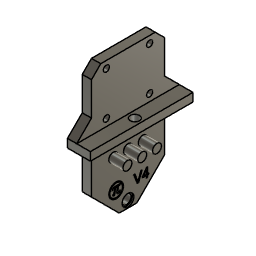
3. BLDC motor holder [V4] (Autodesk Fusion 360 design; units mm, degrees)
Autodesk Fusion 360 part; units mm, degrees
sketch "Base" plane through (0, 0, 0) normal (0, 0, 1) x (1, 0, 0)
  line L0 (0, 0) -> (5, 0)
  line L1 (5, 0) -> (5, 39.5)
  line L2 (5, 39.5) -> (0, 39.5)
  line L3 (0, 39.5) -> (0, 0)
  dimension "d1" = 39.5
  dimension "d2" = 5
  constraint horizontal L0
  constraint vertical L1
  constraint horizontal L2
  constraint vertical L3
  constraint coincident L0.start L3.end
  measures "d1" distance of L0.start L2.end
  measures "d2" distance of L0.start L0.end
extrude "Extrude1" add sketch "Base" along normal blind 39.5 makes body 1
sketch "Bottom round hole" plane through (5, 0, 0) normal (1, 0, 0) x (0, 1, 0)
  circle A0 centre (19.75, 3.7) radius 3.7
  line L0 (0, 0) -> (0, 39.5)
  line L1 (39.5, 0) -> (39.5, 39.5)
  line L2 (39.5, 0) -> (0, 0)
  circle A1 centre (19.75, 3.7) radius 3.2
  circle A2 centre (19.75, 3.7) radius 2.5
  line L3 (0, 0) -> (39.5, 0)
  line L4 (39.5, 0) -> (39.5, 39.5)
  line L5 (39.5, 39.5) -> (0, 39.5)
  line L6 (0, 39.5) -> (0, 0)
  line L7 (24.5, 0) -> (39.5, 15)
  line L8 (24.5, 0) -> (43.435, 0) construction
  line L9 (15, 0) -> (0, 15)
  line L10 (15, 0) -> (21.7279, 0) construction
  dimension "d5" = 19.75
  dimension "d6" = 19.75
  dimension "d7" = 7.4
  dimension "d8" = 6.4
  dimension "d9" = 5
  dimension "d73" = 45
  dimension "d74" = 135
  dimension "d75" = 15
  dimension "d76" = 15
  constraint tangent A0 L2
  constraint concentric A0 A1
  constraint concentric A0 A2
  constraint horizontal L8
  constraint coincident L2 L7.start
  constraint coincident L4 L7.end
  constraint horizontal L10
  constraint coincident L3 L9.start
  constraint coincident L0 L9.end
  measures "d5" distance of A0.centre L0
  measures "d6" distance of A0.centre L1
  measures "d7" diameter of A0
  measures "d8" diameter of A1
  measures "d9" diameter of A2
  measures "d73" angle of L7 L8
  measures "d74" angle of L9 L10
  measures "d75" distance of L1.start L7.start
  measures "d76" distance of L9.start L0.start
sketch "Middle support" plane through (0, 0, 39.5) normal (0, 0, 1) x (-1, 0, 0)
  line L0 (0, -39.5) -> (0, 0)
  line L1 (0, 0) -> (-5, 0)
  line L2 (-5, 0) -> (-5, -39.5)
  line L3 (-5, -39.5) -> (0, -39.5)
  line L4 (0, 8) -> (-13.9, 8)
  line L5 (-13.9, 8) -> (-13.9, -47.5)
  line L6 (-13.9, -47.5) -> (0, -47.5)
  line L7 (0, -47.5) -> (0, 8)
  line L8 (0, 0) -> (-13.9, 0)
  line L9 (-13.9, 0) -> (-13.9, -8)
  line L10 (-13.9, -8) -> (0, -8)
  line L11 (0, -8) -> (0, 0)
  line L12 (0, -39.5) -> (-13.9, -39.5)
  line L13 (-13.9, -39.5) -> (-13.9, -31.5)
  line L14 (-13.9, -31.5) -> (0, -31.5)
  line L15 (0, -31.5) -> (0, -39.5)
  line L16 (0, -39.5) -> (-6.5, -39.5)
  line L17 (-6.5, -39.5) -> (-6.5, -47.5)
  line L18 (-6.5, -47.5) -> (0, -47.5)
  line L19 (0, -47.5) -> (0, -39.5)
  line L20 (0, 0) -> (-6.5, 0)
  line L21 (-6.5, 0) -> (-6.5, 8)
  line L22 (-6.5, 8) -> (0, 8)
  line L23 (0, 8) -> (0, 0)
  dimension "d10" = 13.9
  dimension "d11" = 8
  dimension "d12" = 8
  dimension "d13" = 8
  dimension "d14" = 8
  constraint horizontal L4
  constraint vertical L5
  constraint horizontal L6
  constraint vertical L7
  constraint horizontal L8
  constraint vertical L9
  constraint horizontal L10
  constraint vertical L11
  constraint coincident L5 L9.end
  constraint coincident L0.end L1.start
  constraint horizontal L12
  constraint vertical L13
  constraint horizontal L14
  constraint vertical L15
  constraint coincident L5 L13.end
  constraint coincident L0.start L3.end
  constraint horizontal L16
  constraint vertical L17
  constraint horizontal L18
  constraint vertical L19
  constraint coincident L6 L17.end
  constraint horizontal L20
  constraint vertical L21
  constraint horizontal L22
  constraint vertical L23
  constraint coincident L4 L21.end
  measures "d10" distance of L4.start L4.end
  measures "d11" distance of L3 L6
  measures "d12" distance of L1 L4
  measures "d13" distance of L0.end L10.end
  measures "d14" distance of L0.start L14.end
extrude "Extrude4" add sketch "Middle support" along normal blind 4.5 bodies 1
extrude "Extrude5" add sketch "Middle support" along normal blind 35.5 separate body contours L0 L2 L3 L7 L12 L14 L15 L16 | L0 L2 L7 L10 L14 | L0 L1 L2 L7 L8 L10 L11 L20 makes body 2
sketch "Motor round holes" plane through (5, 0, 0) normal (1, 0, 0) x (0, 1, 0)
  line L0 (0, 39.5) -> (39.5, 39.5)
  line L1 (39.5, 75) -> (0, 75)
  line L2 (19.75, 42.5167) -> (19.75, 75)
  circle A0 centre (8.05, 47.8) radius 3.8
  line L3 (-8, 44) -> (47.5, 44)
  circle A1 centre (8.05, 47.8) radius 1.65
  line L4 (47.5, 44) -> (0, 44)
  line L5 (0, 44) -> (0, 75)
  line L6 (0, 59.5) -> (39.5, 59.5)
  circle A2 centre (8.05, 71.2) radius 1.65
  circle A3 centre (8.05, 71.2) radius 3.8
  circle A4 centre (31.45, 71.2) radius 3.8
  circle A5 centre (31.45, 71.2) radius 1.65
  circle A6 centre (31.45, 47.8) radius 3.8
  circle A7 centre (31.45, 47.8) radius 1.65
  line L7 (39.5, 39.5) -> (39.5, 75)
  line L8 (0, 75) -> (0, 39.5)
  line L9 (0, 75) -> (39.5, 75)
  line L10 (39.5, 75) -> (39.4892, 44)
  dimension "d23" = 11.7
  dimension "d24" = 7.6
  dimension "d25" = 3.3
  constraint midpoint L1 L2.end
  constraint perpendicular L1 L2
  constraint tangent A0 L3
  constraint concentric A0 A1
  constraint horizontal L4
  constraint vertical L5
  constraint coincident L3.end L4.start
  constraint coincident L1.end L5.end
  constraint midpoint L5 L6.start
  constraint symmetric A0 L6 A3
  constraint symmetric A1 L6 A2
  constraint symmetric L2 A0 A6
  constraint symmetric L2 A1 A7
  constraint symmetric L2 A2 A5
  constraint symmetric L2 A3 A4
  constraint coincident L1.start L7.end
  constraint coincident L4 L10.end
  constraint coincident L6.end L7
  constraint perpendicular L6 L7
  measures "d23" distance of L2 A0.centre
  measures "d24" diameter of A0
  measures "d25" diameter of A1
sketch "Middle top round hole" plane through (0, 0, 39.5) normal (0, 0, 1) x (-1, 0, 0)
  line L0 (-5, -8) -> (-12.4, -8)
  line L1 (-12.4, -8) -> (-12.4, -31.5)
  line L2 (-12.4, -31.5) -> (-5, -31.5)
  line L3 (-5, -31.5) -> (-5, -8)
  line L4 (-12.4, -19.75) -> (-5, -19.75)
  line L5 (-8.7, -8) -> (-8.7, -31.5)
  circle A0 centre (-8.7, -19.75) radius 3.2
  circle A1 centre (-8.7, -19.75) radius 2.5
  dimension "d26" = 6.4
  dimension "d27" = 5
  constraint horizontal L0
  constraint vertical L1
  constraint horizontal L2
  constraint vertical L3
  constraint midpoint L1 L4.start
  constraint midpoint L3 L4.end
  constraint midpoint L0 L5.start
  constraint midpoint L2 L5.end
  constraint midpoint L4 A0.centre
  constraint concentric A0 A1
  measures "d26" diameter of A0
  measures "d27" diameter of A1
extrude "Extrude6" cut sketch "Middle top round hole" along normal blind 5 contours L4 L5 A1 | L4 L5 A1 | L4 L5 A1 | L4 L5 A1 bodies 1
extrude "Extrude7" cut sketch "Middle top round hole" along normal blind 0.8 contours L4 L5 A0 A1 | L4 L5 A0 A1 | L4 L5 A0 A1 | L4 L5 A0 A1 bodies 1
extrude "Extrude8" cut sketch "Motor round holes" against normal blind 7 contours A1 | A2 | A5 | A7 bodies 2
extrude "Extrude9" cut sketch "Bottom round hole" against normal blind 10 contours A2 bodies 1
extrude "Extrude10" cut sketch "Bottom round hole" against normal blind 0.8 contours A1 bodies 1
extrude "Extrude11" add 1 faces at (4.2, 22.6954, 3.4168) along direction (-1, 0, 0) blind 6.1 on bodies 1 bodies 1
extrude "Extrude12" add sketch "Bottom round hole" against normal blind 7.7 contours A0 bodies 1
sketch "Motor rest area support" plane through (0, 0, 0) normal (-1, 0, 0) x (0, -1, 0)
  circle A0 centre (-31.45, 71.2) radius 1.65
  circle A1 centre (-8.05, 47.8) radius 1.65
  circle A2 centre (-8.05, 71.2) radius 1.65
  circle A3 centre (-31.45, 47.8) radius 1.65
  line L0 (-39.5, 39.5) -> (0, 39.5)
  line L1 (0, 39.5) -> (0, 75)
  line L2 (0, 75) -> (-39.5, 75)
  line L3 (-39.5, 75) -> (-39.5, 39.5)
  line L4 (-47.5, 44) -> (-39.5, 52)
  line L5 (-47.5, 44) -> (-36.1863, 44) construction
  line L6 (8, 44) -> (0, 52)
  line L7 (8, 44) -> (19.3137, 44) construction
  line L8 (0, 52) -> (8, 52)
  line L9 (8, 52) -> (8, 44)
  line L10 (8, 44) -> (0, 44)
  line L11 (0, 44) -> (0, 52)
  line L12 (-39.5, 52) -> (-47.5, 52)
  line L13 (-47.5, 52) -> (-47.5, 44)
  line L14 (-47.5, 44) -> (-39.5, 44)
  line L15 (-39.5, 44) -> (-39.5, 52)
  line L16 (-5, 75) -> (0, 70)
  line L17 (-5, 75) -> (2.4834, 75) construction
  line L18 (-34.5, 75) -> (-39.5, 70)
  line L19 (-34.5, 75) -> (-27.8923, 75) construction
  dimension "d42" = 45
  dimension "d43" = 135
  dimension "d67" = 45
  dimension "d68" = 5
  dimension "d69" = 135
  dimension "d70" = 5
  constraint horizontal L5
  constraint coincident L3 L4.end
  constraint horizontal L7
  constraint coincident L1 L6.end
  constraint horizontal L8
  constraint vertical L9
  constraint horizontal L10
  constraint vertical L11
  constraint horizontal L12
  constraint vertical L13
  constraint horizontal L14
  constraint vertical L15
  constraint horizontal L17
  constraint coincident L2 L16.start
  constraint coincident L1 L16.end
  constraint horizontal L19
  constraint coincident L2 L18.start
  constraint coincident L3 L18.end
  measures "d42" angle of L4 L5
  measures "d43" angle of L6 L7
  measures "d67" angle of L16 L17
  measures "d68" distance of L1.end L16.start
  measures "d69" angle of L18 L19
  measures "d70" distance of L2.end L18.start
extrude "Extrude13" add sketch "Motor rest area support" against normal blind 5 contours L3 L4 L14 L15 | L1 L6 L10 L11 bodies 1 2
sketch "Middle round holes" plane through (5, 0, 0) normal (1, 0, 0) x (0, 1, 0)
  circle A0 centre (19.75, 3.7) radius 3.2
  line L0 (0, 0) -> (39.5, 0)
  line L1 (39.5, 0) -> (39.5, 39.5)
  line L2 (39.5, 39.5) -> (0, 39.5)
  line L3 (0, 39.5) -> (0, 0)
  line L4 (0, 31.5) -> (39.5, 31.5) construction
  line L5 (0, 24.1) -> (39.5, 24.1) construction
  line L6 (19.75, 31.5) -> (19.75, 24)
  line L7 (19.75, 27.75) -> (39.5, 27.75)
  line L8 (19.75, 27.75) -> (0, 27.75)
  circle A1 centre (19.75, 27.75) radius 2.425
  circle A2 centre (19.75, 27.75) radius 3.2
  circle A3 centre (27.75, 27.75) radius 2.425
  circle A4 centre (27.75, 27.75) radius 3.2
  circle A5 centre (11.75, 27.75) radius 2.425
  circle A6 centre (11.75, 27.75) radius 3.2
  dimension "d46" = 8
  dimension "d47" = 7.4
  dimension "d48" = 6.4
  dimension "d49" = 4.85
  dimension "d52" = 8
  dimension "d53" = 0
  dimension "d56" = -8
  dimension "d57" = 0
  constraint coincident L3 L4.start
  constraint coincident L1 L4.end
  constraint perpendicular L1 L4
  constraint coincident L1 L5.end
  constraint perpendicular L1 L5
  constraint midpoint L4 L6.start
  constraint perpendicular L4 L6
  constraint midpoint L6 L7.start
  constraint coincident L1 L7.end
  constraint perpendicular L1 L7
  constraint coincident L3 L8.end
  constraint perpendicular L3 L8
  constraint coincident L7.start L8.start
  constraint concentric A1 A2
  measures "d46" distance of L2 L4
  measures "d47" distance of L4 L5
  measures "d48" diameter of A2
  measures "d49" diameter of A1
extrude "Extrude14" add sketch "Middle round holes" along normal blind 7.7 contours L8 A5 | L8 A5 | L7 A3 | L7 A3 | L6 L8 A1 | L6 L8 A1 | L6 L7 A1 | L6 L7 A1 bodies 1
sketch "Author" plane through (5, 0, 0) normal (1, 0, 0) x (0, 1, 0)
  circle A0 centre (27.75, 27.75) radius 2.425
  circle A1 centre (19.75, 27.75) radius 2.425
  circle A2 centre (11.75, 27.75) radius 2.425
  circle A3 centre (19.75, 3.7) radius 3.2
  line L0 (0, 0) -> (39.5, 0)
  line L1 (39.5, 0) -> (39.5, 39.5)
  line L2 (39.5, 39.5) -> (0, 39.5)
  line L3 (0, 39.5) -> (0, 0)
  line L4 (11.1685, 12.3321) -> (11.3277, 12.3203)
  spline S0 degree 3 poles (11.3277, 12.3203) (11.4928, 12.507) (11.5577, 13.0594) (12.5307, 12.9513) knots 0 0 0 0 1 1 1 1
  spline S1 degree 3 poles (12.5307, 12.9513) (12.4953, 10.5845) (11.4574, 10.3348) (11.5223, 9.8493) knots 0 0 0 0 1 1 1 1
  spline S2 degree 3 poles (11.5223, 9.8493) (11.5459, 9.5741) (11.7641, 9.405) (12, 9.3952) knots 0 0 0 0 1 1 1 1
  spline S3 degree 3 poles (12, 9.3952) (12.745, 9.4208) (12.7116, 10.4253) (12.9435, 12.9572) knots 0 0 0 0 1 1 1 1
  line L5 (12.9435, 12.9572) -> (13.9048, 12.9572)
  spline S4 degree 3 poles (13.9048, 12.9572) (13.8537, 12.0647) (13.7141, 11.1723) (13.6984, 10.2975) knots 0 0 0 0 1 1 1 1
  spline S5 degree 3 poles (13.6984, 10.2975) (13.7102, 9.7156) (14.064, 9.405) (14.5299, 9.4011) knots 0 0 0 0 1 1 1 1
  spline S6 degree 3 poles (14.5299, 9.4011) (15.2965, 9.3756) (15.5383, 10.27) (15.5383, 10.6513) knots 0 0 0 0 1 1 1 1
  line L6 (15.5383, 10.6513) -> (15.3732, 10.6513)
  spline S7 degree 3 poles (15.3732, 10.6513) (15.3575, 10.3368) (15.2061, 10.1107) (14.8837, 10.097) knots 0 0 0 0 1 1 1 1
  spline S8 degree 3 poles (14.8837, 10.097) (14.005, 10.0852) (14.4886, 11.6421) (14.4945, 12.9454) knots 0 0 0 0 1 1 1 1
  line L7 (14.4945, 12.9454) -> (15.5383, 12.9395)
  line L8 (15.5383, 12.9395) -> (15.5324, 13.6059)
  spline S9 degree 3 poles (15.5324, 13.6059) (11.1939, 13.6269) (11.7446, 13.7119) (11.1685, 12.3321) knots 0 0 0 0 1 1 1 1
  arc A4 (9.3808, 11.5049) -> (13.3534, 15.4775) centre (13.3534, 11.5049) cw
  arc A5 (13.3534, 7.5323) -> (9.3808, 11.5049) centre (13.3534, 11.5049) cw
  arc A6 (17.326, 11.5049) -> (13.3534, 7.5323) centre (13.3534, 11.5049) cw
  arc A7 (13.3534, 15.4775) -> (17.326, 11.5049) centre (13.3534, 11.5049) cw
  arc A8 (13.3534, 14.9461) -> (13.442, 14.945) centre (13.3538, 11.5049) cw
  arc A9 (13.442, 14.945) -> (13.5306, 14.9415) centre (13.3532, 11.5049) cw
  arc A10 (13.5306, 14.9415) -> (13.619, 14.9358) centre (13.3531, 11.5049) cw
  arc A11 (13.619, 14.9358) -> (13.7072, 14.9279) centre (13.3538, 11.5049) cw
  arc A12 (13.7072, 14.9279) -> (13.7952, 14.9176) centre (13.3534, 11.5049) cw
  arc A13 (13.7952, 14.9176) -> (13.883, 14.9051) centre (13.3536, 11.5049) cw
  arc A14 (13.883, 14.9051) -> (13.9703, 14.8903) centre (13.3527, 11.505) cw
  arc A15 (13.9703, 14.8903) -> (14.0573, 14.8733) centre (13.3537, 11.5049) cw
  arc A16 (14.0573, 14.8733) -> (14.1438, 14.8541) centre (13.3537, 11.5049) cw
  arc A17 (14.1438, 14.8541) -> (14.2298, 14.8326) centre (13.3528, 11.5051) cw
  arc A18 (14.2298, 14.8326) -> (14.3152, 14.809) centre (13.3542, 11.5047) cw
  arc A19 (14.3152, 14.809) -> (14.3999, 14.7831) centre (13.353, 11.505) cw
  arc A20 (14.3999, 14.7831) -> (14.484, 14.7551) centre (13.3531, 11.505) cw
  arc A21 (14.484, 14.7551) -> (14.5673, 14.7249) centre (13.3537, 11.5048) cw
  arc A22 (14.5673, 14.7249) -> (14.6498, 14.6925) centre (13.353, 11.5051) cw
  arc A23 (14.6498, 14.6925) -> (14.7314, 14.6581) centre (13.3537, 11.5048) cw
  arc A24 (14.7314, 14.6581) -> (14.8122, 14.6216) centre (13.3537, 11.5048) cw
  arc A25 (14.8122, 14.6216) -> (14.8919, 14.583) centre (13.3532, 11.505) cw
  arc A26 (14.8919, 14.583) -> (14.9707, 14.5424) centre (13.3537, 11.5048) cw
  arc A27 (14.9707, 14.5424) -> (15.0483, 14.4997) centre (13.3529, 11.5052) cw
  arc A28 (15.0483, 14.4997) -> (15.1249, 14.4551) centre (13.3536, 11.5048) cw
  arc A29 (15.1249, 14.4551) -> (15.2003, 14.4085) centre (13.3533, 11.505) cw
  arc A30 (15.2003, 14.4085) -> (15.2744, 14.36) centre (13.3532, 11.505) cw
  arc A31 (15.2744, 14.36) -> (15.3473, 14.3096) centre (13.3537, 11.5047) cw
  arc A32 (15.3473, 14.3096) -> (15.4188, 14.2573) centre (13.3536, 11.5048) cw
  arc A33 (15.4188, 14.2573) -> (15.489, 14.2032) centre (13.3531, 11.5052) cw
  arc A34 (15.489, 14.2032) -> (15.5578, 14.1473) centre (13.3535, 11.5048) cw
  arc A35 (15.5578, 14.1473) -> (15.6251, 14.0897) centre (13.3533, 11.505) cw
  arc A36 (15.6251, 14.0897) -> (15.6909, 14.0303) centre (13.3533, 11.505) cw
  arc A37 (15.6909, 14.0303) -> (15.7551, 13.9693) centre (13.3537, 11.5046) cw
  arc A38 (15.7551, 13.9693) -> (15.8178, 13.9067) centre (13.3534, 11.5049) cw
  arc A39 (15.8178, 13.9067) -> (15.8788, 13.8424) centre (13.3531, 11.5053) cw
  arc A40 (15.8788, 13.8424) -> (15.9382, 13.7766) centre (13.3535, 11.5048) cw
  arc A41 (15.9382, 13.7766) -> (15.9958, 13.7093) centre (13.3535, 11.5049) cw
  arc A42 (15.9958, 13.7093) -> (16.0517, 13.6405) centre (13.3533, 11.5051) cw
  arc A43 (16.0517, 13.6405) -> (16.1058, 13.5704) centre (13.3536, 11.5046) cw
  arc A44 (16.1058, 13.5704) -> (16.158, 13.4988) centre (13.3532, 11.5052) cw
  arc A45 (16.158, 13.4988) -> (16.2084, 13.4259) centre (13.3532, 11.5052) cw
  arc A46 (16.2084, 13.4259) -> (16.257, 13.3518) centre (13.3535, 11.5048) cw
  arc A47 (16.257, 13.3518) -> (16.3036, 13.2764) centre (13.3535, 11.5048) cw
  arc A48 (16.3036, 13.2764) -> (16.3482, 13.1999) centre (13.3533, 11.5051) cw
  arc A49 (16.3482, 13.1999) -> (16.3908, 13.1222) centre (13.3537, 11.5044) cw
  arc A50 (16.3908, 13.1222) -> (16.4315, 13.0434) centre (13.3532, 11.5052) cw
  arc A51 (16.4315, 13.0434) -> (16.4701, 12.9637) centre (13.3535, 11.5047) cw
  arc A52 (16.4701, 12.9637) -> (16.5066, 12.883) centre (13.3533, 11.5052) cw
  arc A53 (16.5066, 12.883) -> (16.541, 12.8013) centre (13.3536, 11.5045) cw
  arc A54 (16.541, 12.8013) -> (16.5734, 12.7188) centre (13.3533, 11.5053) cw
  arc A55 (16.5734, 12.7188) -> (16.6035, 12.6355) centre (13.3533, 11.5052) cw
  arc A56 (16.6035, 12.6355) -> (16.6316, 12.5514) centre (13.3535, 11.5046) cw
  arc A57 (16.6316, 12.5514) -> (16.6574, 12.4667) centre (13.3535, 11.5045) cw
  arc A58 (16.6574, 12.4667) -> (16.6811, 12.3813) centre (13.3532, 11.5057) cw
  arc A59 (16.6811, 12.3813) -> (16.7026, 12.2953) centre (13.3535, 11.5043) cw
  arc A60 (16.7026, 12.2953) -> (16.7218, 12.2088) centre (13.3533, 11.5052) cw
  arc A61 (16.7218, 12.2088) -> (16.7388, 12.1219) centre (13.3535, 11.5045) cw
  arc A62 (16.7388, 12.1219) -> (16.7536, 12.0345) centre (13.3534, 11.505) cw
  arc A63 (16.7536, 12.0345) -> (16.7661, 11.9468) centre (13.3534, 11.5051) cw
  arc A64 (16.7661, 11.9468) -> (16.7763, 11.8588) centre (13.3534, 11.5049) cw
  arc A65 (16.7763, 11.8588) -> (16.7843, 11.7705) centre (13.3534, 11.5053) cw
  arc A66 (16.7843, 11.7705) -> (16.79, 11.6821) centre (13.3534, 11.5047) cw
  arc A67 (16.79, 11.6821) -> (16.7934, 11.5935) centre (13.3534, 11.5047) cw
  arc A68 (16.7934, 11.5935) -> (16.7946, 11.5049) centre (13.3534, 11.5054) cw
  arc A69 (16.7946, 11.5049) -> (16.7849, 11.2478) centre (13.3534, 11.5047) cw
  arc A70 (16.7849, 11.2478) -> (16.7561, 10.992) centre (13.3534, 11.505) cw
  arc A71 (16.7561, 10.992) -> (16.7083, 10.7392) centre (13.3534, 11.5048) cw
  arc A72 (16.7083, 10.7392) -> (16.6417, 10.4906) centre (13.3534, 11.505) cw
  arc A73 (16.6417, 10.4906) -> (16.5567, 10.2477) centre (13.3534, 11.505) cw
  arc A74 (16.5567, 10.2477) -> (16.4538, 10.0119) centre (13.3534, 11.5049) cw
  arc A75 (16.4538, 10.0119) -> (16.3335, 9.7843) centre (13.3533, 11.5048) cw
  arc A76 (16.3335, 9.7843) -> (16.1966, 9.5665) centre (13.3534, 11.505) cw
  arc A77 (16.1966, 9.5665) -> (16.0438, 9.3594) centre (13.3534, 11.505) cw
  arc A78 (16.0438, 9.3594) -> (15.8759, 9.1643) centre (13.3534, 11.5049) cw
  arc A79 (15.8759, 9.1643) -> (15.694, 8.9824) centre (13.3533, 11.5048) cw
  arc A80 (15.694, 8.9824) -> (15.4989, 8.8145) centre (13.3536, 11.5051) cw
  arc A81 (15.4989, 8.8145) -> (15.2919, 8.6617) centre (13.3534, 11.5049) cw
  arc A82 (15.2919, 8.6617) -> (15.074, 8.5248) centre (13.3534, 11.505) cw
  arc A83 (15.074, 8.5248) -> (14.8465, 8.4045) centre (13.3534, 11.5049) cw
  arc A84 (14.8465, 8.4045) -> (14.6106, 8.3016) centre (13.3534, 11.5049) cw
  arc A85 (14.6106, 8.3016) -> (14.3677, 8.2166) centre (13.3534, 11.5049) cw
  arc A86 (14.3677, 8.2166) -> (14.1191, 8.15) centre (13.3532, 11.5049) cw
  arc A87 (14.1191, 8.15) -> (13.8663, 8.1022) centre (13.3535, 11.5049) cw
  arc A88 (13.8663, 8.1022) -> (13.6106, 8.0734) centre (13.3533, 11.5049) cw
  arc A89 (13.6106, 8.0734) -> (13.3534, 8.0638) centre (13.3536, 11.5049) cw
  arc A90 (13.3534, 8.0638) -> (13.0962, 8.0734) centre (13.3532, 11.5049) cw
  arc A91 (13.0962, 8.0734) -> (12.8405, 8.1022) centre (13.3535, 11.5049) cw
  arc A92 (12.8405, 8.1022) -> (12.5877, 8.15) centre (13.3533, 11.5049) cw
  arc A93 (12.5877, 8.15) -> (12.3391, 8.2166) centre (13.3535, 11.5049) cw
  arc A94 (12.3391, 8.2166) -> (12.0962, 8.3016) centre (13.3534, 11.5049) cw
  arc A95 (12.0962, 8.3016) -> (11.8603, 8.4045) centre (13.3534, 11.5049) cw
  arc A96 (11.8603, 8.4045) -> (11.6328, 8.5248) centre (13.3534, 11.5049) cw
  arc A97 (11.6328, 8.5248) -> (11.4149, 8.6617) centre (13.3534, 11.505) cw
  arc A98 (11.4149, 8.6617) -> (11.2079, 8.8145) centre (13.3534, 11.5049) cw
  arc A99 (11.2079, 8.8145) -> (11.0128, 8.9824) centre (13.3532, 11.5051) cw
  arc A100 (11.0128, 8.9824) -> (10.8308, 9.1643) centre (13.3534, 11.5049) cw
  arc A101 (10.8308, 9.1643) -> (10.663, 9.3594) centre (13.3535, 11.5047) cw
  arc A102 (10.663, 9.3594) -> (10.5102, 9.5665) centre (13.3534, 11.505) cw
  arc A103 (10.5102, 9.5665) -> (10.3733, 9.7843) centre (13.3533, 11.505) cw
  arc A104 (10.3733, 9.7843) -> (10.253, 10.0119) centre (13.3535, 11.5048) cw
  arc A105 (10.253, 10.0119) -> (10.1501, 10.2477) centre (13.3534, 11.5049) cw
  arc A106 (10.1501, 10.2477) -> (10.0651, 10.4906) centre (13.3534, 11.505) cw
  arc A107 (10.0651, 10.4906) -> (9.9985, 10.7392) centre (13.3534, 11.505) cw
  arc A108 (9.9985, 10.7392) -> (9.9507, 10.992) centre (13.3534, 11.5048) cw
  arc A109 (9.9507, 10.992) -> (9.9218, 11.2478) centre (13.3534, 11.505) cw
  arc A110 (9.9218, 11.2478) -> (9.9122, 11.5049) centre (13.3534, 11.5047) cw
  arc A111 (9.9122, 11.5049) -> (9.9218, 11.7621) centre (13.3534, 11.5051) cw
  arc A112 (9.9218, 11.7621) -> (9.9507, 12.0178) centre (13.3534, 11.5048) cw
  arc A113 (9.9507, 12.0178) -> (9.9985, 12.2706) centre (13.3534, 11.505) cw
  arc A114 (9.9985, 12.2706) -> (10.0651, 12.5192) centre (13.3533, 11.5047) cw
  arc A115 (10.0651, 12.5192) -> (10.1501, 12.7621) centre (13.3534, 11.505) cw
  arc A116 (10.1501, 12.7621) -> (10.253, 12.998) centre (13.3534, 11.5049) cw
  arc A117 (10.253, 12.998) -> (10.3733, 13.2255) centre (13.3534, 11.5049) cw
  arc A118 (10.3733, 13.2255) -> (10.5102, 13.4434) centre (13.3534, 11.505) cw
  arc A119 (10.5102, 13.4434) -> (10.663, 13.6505) centre (13.3534, 11.5049) cw
  arc A120 (10.663, 13.6505) -> (10.8308, 13.8455) centre (13.3535, 11.5051) cw
  arc A121 (10.8308, 13.8455) -> (11.0128, 14.0275) centre (13.3533, 11.5048) cw
  arc A122 (11.0128, 14.0275) -> (11.2079, 14.1953) centre (13.3534, 11.5049) cw
  arc A123 (11.2079, 14.1953) -> (11.4149, 14.3482) centre (13.3534, 11.5049) cw
  arc A124 (11.4149, 14.3482) -> (11.6328, 14.4851) centre (13.3534, 11.5049) cw
  arc A125 (11.6328, 14.4851) -> (11.8603, 14.6053) centre (13.3534, 11.5049) cw
  arc A126 (11.8603, 14.6053) -> (12.0962, 14.7082) centre (13.3534, 11.5049) cw
  arc A127 (12.0962, 14.7082) -> (12.3391, 14.7932) centre (13.3534, 11.5049) cw
  arc A128 (12.3391, 14.7932) -> (12.5877, 14.8598) centre (13.3535, 11.505) cw
  arc A129 (12.5877, 14.8598) -> (12.8405, 14.9077) centre (13.3533, 11.5049) cw
  arc A130 (12.8405, 14.9077) -> (13.0962, 14.9365) centre (13.3535, 11.5049) cw
  arc A131 (13.0962, 14.9365) -> (13.3534, 14.9461) centre (13.3532, 11.5049) cw
  dimension "d60" = 9.3808
  dimension "d61" = 7.5323
  measures "d60" distance of L3 A4.start
  measures "d61" distance of L0 A5.start
sketch "Version" plane through (5, 0, 0) normal (1, 0, 0) x (0, 1, 0)
  line L0 (22.826, 9.0323) -> (31.5, 9.0323) construction
  line L1 (31.5, 9.0323) -> (31.5, 14.0323) construction
  line L2 (31.5, 14.0323) -> (22.826, 14.0323) construction
  line L3 (22.826, 14.0323) -> (22.826, 9.0323) construction
  point P0 (17.326, 11.5049)
  point P1 (13.3534, 7.5323)
  dimension "d62" = 5
  dimension "d63" = 5.5
  dimension "d64" = 1.5
  text T0 "V4" font "Arial" height 5 align left top in box 8.674 x 5 at (22.826, 9.0323) x (1, 0) y (0, 1) spacing 1 kerned
  measures "d63" distance of P0
  measures "d64" distance of L0 P1
extrude "Extrude15" cut sketch "Author" sketch "Version" against normal blind 1 contours L4 S0 S1 S2 S3 L5 S4 S5 S6 L6 S7 S8 L7 L8 S9 | A4 A5 A6 A7 of sketch 2 text T0 bodies 1
extrude "Extrude16" cut sketch "Motor rest area support" against normal blind 7 contours L2 L3 L18 | L1 L2 L16 bodies 1
extrude "Extrude17" cut sketch "Bottom round hole" against normal blind 7 contours L1 L2 L3 L4 L7 | L0 L2 L3 L6 L9 bodies 1
extrude "Extrude18" cut 1 faces at (13.9, 10.5, 41) along direction (-1, 0, 0) blind 1.5 on bodies 1 bodies 1
named bodies: "Base", "Motor rest area"
